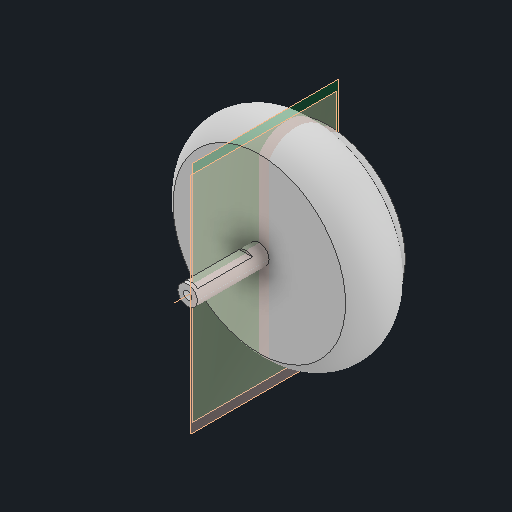
# Autodesk Inventor part: Wheel
Saved by Autodesk Inventor 2027 (Build 310192000, 192)
## iProperties
Created: 2026-07-06
Part Number: Wheel
Material: Generic
Document SubType Name: Modeling
Designer: belcz
Density: 1 g/cm^3
Appearance: Default
Author: belcz
Autodesk Inventor part; units mm, degrees
ref_plane "XZ Plane" through (0, 0, 0) normal (0, 1, 0) x (-1, 0, 0)
ref_plane "XY Plane" through (0, 0, 0) normal (0, 0, 1) x (1, 0, 0)
sketch "Sketch1" plane through (0, 0, 0) normal (0, 0, 1) x (1, 0, 0)
  circle A0 centre (0, 0) radius 7.9375
  dimension "d0" = 15.875
  constraints: 1 centre point, 1 coincident
  measures "d0" diameter of A0
extrude "Extrusion1" add sketch "Sketch1" along normal blind 58.039
sketch "Sketch2" plane through (0, 0, 0) normal (0, 0, -1) x (-1, 0, 0)
  circle A0 centre (0, 0) radius 82.55
  dimension "d3" = 165.1
  constraints: 1 centre point, 1 coincident
  measures "d3" diameter of A0
extrude "Extrusion2" add sketch "Sketch2" along normal blind 45.4533
sketch "Sketch3" plane through (0, 0, -45.4533) normal (0, 0, -1) x (-1, 0, 0)
  circle A0 centre (0, 0) radius 67.2719
  circle A1 centre (0, 0) radius 53.975
  dimension "d6" = 134.5438
  dimension "d20" = 107.95
  constraints: 2 centre point, 2 coincident
  measures "d6" diameter of A0
  measures "d20" diameter of A1
ref_plane "Work Plane3" through (0, 0, -45.4533) normal (0, 0, -1) x (-1, 0, 0)
sketch "Sketch4" plane through (0, 0, -45.4533) normal (0, 0, -1) x (-1, 0, 0)
  point P0 (0, 0)
ref_plane "Work Plane1" through (7.9375, 0, 0) normal (1, 0, 0) x (0, 1, 0)
sketch "Sketch5" plane through (7.9375, 0, 0) normal (1, 0, 0) x (0, 1, 0)
  line L0 (-7.9375, 0) -> (-7.9375, 58.039) projected
  line L1 (7.9375, 58.039) -> (-7.9375, 58.039) projected
  line L2 (7.9375, 58.039) -> (-7.9375, 58.039) projected
  line L3 (7.9375, 0) -> (-7.9375, 0) projected
  line L4 (7.9375, 0) -> (7.9375, 58.039) projected
  line L5 (5.8928, 55.245) -> (5.8928, 10.8077)
  line L6 (5.8928, 55.245) -> (7.9375, 55.245)
  line L7 (5.8928, 10.8077) -> (7.9375, 10.8077)
  point P0 (0, 0)
  dimension "d9" = 13.8303
  dimension "d10" = 2.794
  dimension "d11" = 10.8077
  constraints: 6 end point, 2 perpendicular, 2 point on line, 1 vertical
  measures "d9" distance between parallel lines of L0 L5
  measures "d10" distance between parallel lines of L1 L6
  measures "d11" distance between parallel lines of L3 L7
extrude "Extrusion4" cut sketch "Sketch5" against normal blind 50.8 contours L7 L5 L6 L4
sketch "Sketch6" plane through (0, 0, 58.039) normal (0, 0, 1) x (1, 0, 0)
  circle A0 centre (0, 0) radius 3.2512
  dimension "d14" = 6.5024
  constraints: 1 centre point, 1 coincident
  measures "d14" diameter of A0
ref_plane "Work Plane2" through (0, 0, -49.2633) normal (-1, 0, 0) x (0, 0, 1)
extrude "Extrusion6" add sketch "Sketch3" along normal blind 10.16 draft -25
extrude "Extrusion7" add sketch "Sketch3" along normal blind 10.16 draft 25 contours A1
sketch "Sketch8" plane through (0, 0, -49.2633) normal (-1, 0, 0) x (0, 0, 1)
  line L0 (49.2633, 82.55) -> (3.81, 82.55) projected
  line L1 (26.5367, 82.55) -> (26.5367, 46.429)
  arc A0 (49.2633, 69.85) -> (26.5367, 82.55) centre (26.5367, 55.8653) ccw
  line L2 (49.2633, 82.55) -> (49.2633, -82.55) projected
  arc A1 (26.5367, 82.55) -> (3.81, 69.85) centre (26.5367, 55.8653) ccw
  line L3 (49.2633, 82.55) -> (3.81, 82.55) projected
  line L4 (3.81, 82.55) -> (3.81, -82.55) projected
  line L5 (-29.0805, 0) -> (130.0328, 0) projected
  point P0 (49.2633, 0)
  dimension "d25" = 0
  dimension "d26" = 12.7
  constraints: 4 point on circle, 2 centre point, 2 end point, 1 midpoint, 1 symmetric about line, 1 tangent, 1 vertical, 1 other
  measures "d25" distance from line of L2 A0.start
  measures "d26" distance from line of L0 A0.start
revolve "Revolution2" cut sketch "Sketch8" angle 360 about axis through (0, 0, -49.2633) along (0, 0, 1) contours L2 A0 L0 | A1 L4 L0
extrude "Extrusion8" cut sketch "Sketch6" against normal blind 50.8
body "Solid1"
